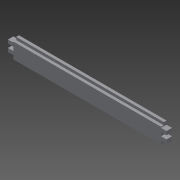
# Autodesk Inventor part: top_cover_side
Saved by Autodesk Inventor 2014 SP1 (Build 180222100, 222)
## iProperties
Created: 2014-02-23
Part Number: top_cover_side
Material: Wood (Birch)
Document SubType Name: Modeling
Designer: Chris
Density: 0.55 g/cm^3
Appearance: Birch - Natural Polished
Mass: 326.682 g
Surface Area: 919.958 cm^2
Volume: 593.967 cm^3
Author: Chris
Autodesk Inventor part; units mm, degrees
ref_plane "YZ Plane" through (0, 0, 0) normal (1, 0, 0) x (0, 1, 0)
ref_plane "XZ Plane" through (0, 0, 0) normal (0, 1, 0) x (-1, 0, 0)
ref_plane "XY Plane" through (0, 0, 0) normal (0, 0, 1) x (1, 0, 0)
sketch "Sketch1" plane through (0, 0, 0) normal (0, 0, 1) x (1, 0, 0)
  line L0 (266.7, 89.6306) -> (523.875, 89.6306)
  line L1 (523.875, 89.6306) -> (523.875, 26.1306)
  line L2 (523.875, 26.1306) -> (266.7, 26.1306)
  line L3 (266.7, 89.6306) -> (266.7, 76.9306)
  line L4 (266.7, 76.9306) -> (247.65, 76.9306)
  line L5 (247.65, 76.9306) -> (247.65, 64.2306)
  line L6 (247.65, 64.2306) -> (266.7, 64.2306)
  line L7 (266.7, 64.2306) -> (266.7, 51.5306)
  line L8 (266.7, 51.5306) -> (247.65, 51.5306)
  line L9 (247.65, 51.5306) -> (247.65, 38.8306)
  line L10 (247.65, 38.8306) -> (266.7, 38.8306)
  line L11 (266.7, 38.8306) -> (266.7, 26.1306)
  point P0 (0, 0)
  dimension "d4" = 63.5
  dimension "d17" = 257.175
  dimension "d18" = 19.05
  dimension "d19" = 12.7
  dimension "d20" = 12.7
  dimension "d21" = 12.7
  dimension "d22" = 12.7
  dimension "d23" = 12.7
  dimension "d24" = 0
  constraints: 24 end point, 7 perpendicular, 4 parallel, 1 horizontal
  measures "d4" distance of L0.end L1.end
  measures "d17" distance of L0.start L0.end
  measures "d18" distance of L3.end L4.end
  measures "d19" distance of L0.start L3.end
  measures "d20" distance of L4.end L5.end
  measures "d21" distance of L6.end L7.end
  measures "d22" distance of L8.end L9.end
  measures "d23" distance of L10.end L2.end
  measures "d24" distance between parallel lines of L11 L7
extrude "Extrusion1" add sketch "Sketch1" along normal blind 19.05
mirror "Mirror1" about plane through (523.875, 26.1306, 0) normal (1, 0, 0) of "Extrusion1"
sketch "Sketch3" plane through (0, 0, 19.05) normal (0, 0, 1) x (1, 0, 0)
  line L0 (266.7, 89.6306) -> (781.05, 89.6306)
  line L1 (781.05, 89.6306) -> (781.05, 80.1056)
  line L2 (781.05, 80.1056) -> (266.7, 80.1056)
  line L3 (266.7, 80.1056) -> (266.7, 89.6306)
  point P0 (0, 0)
  dimension "d25" = 9.525
  constraints: 8 end point, 2 parallel, 1 horizontal, 1 perpendicular
  measures "d25" distance between parallel lines of L0 L2
extrude "Extrusion3" cut sketch "Sketch3" against normal blind 9.525
body "Solid1"
